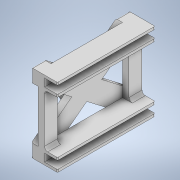
# Autodesk Inventor part: New_ThinGripper
Saved by Autodesk Inventor 2021 (Build 250183000, 183)
## iProperties
Created: 2021-08-05
Part Number: New_ThinGripper
Material: Generic
Document SubType Name: Modeling
Designer: hp
Density: 1 g/cm^3
Appearance: Default
Author: hp
Autodesk Inventor part; units mm, degrees
sketch "Sketch1" plane through (0, 0, 0) normal (1, 0, 0) x (0, 1, 0)
  circle A0 centre (0, 0) radius 2.5
  dimension "d0" = 5
  constraints: 1 centre point, 1 coincident
  measures "d0" diameter of A0
extrude "Extrusion1" add sketch "Sketch1" along normal blind 1
ref_plane "Work Plane1" through (1, 0, 0) normal (1, 0, 0) x (0, 0, -1)
sketch "Sketch2" plane through (1, 0, 0) normal (1, 0, 0) x (0, 0, -1)
  line L0 (-7.5, -6) -> (7.5, -6)
  line L1 (7.5, -6) -> (7.5, 6)
  line L2 (7.5, 6) -> (-7.5, 6)
  line L3 (-7.5, 6) -> (-7.5, -6)
  line L4 (-7.5, -6) -> (7.5, 6) construction
  line L5 (7.5, -6) -> (-7.5, 6) construction
  line L6 (7.5, 6) -> (5.5, 6)
  line L7 (7.5, 6) -> (7.5, 4)
  line L8 (7.5, -6) -> (7.5, -4)
  line L9 (7.5, -6) -> (5.5, -6)
  line L10 (-7.5, -6) -> (-5.5, -6)
  line L11 (-7.5, 6) -> (-7.5, 4)
  line L12 (-7.5, 6) -> (-5.5, 6)
  line L13 (-7.5, -6) -> (-7.5, -4)
  line L14 (-7.5, -4) -> (5.5, 6)
  line L15 (-5.5, -6) -> (7.5, 4)
  line L16 (-5.5, 6) -> (7.5, -4)
  line L17 (-7.5, 4) -> (5.5, -6)
  point P0 (0, 0)
  point P1 (-2.3, 0)
  point P2 (0, -1.7692)
  point P3 (2.3, 0)
  point P4 (0, 1.7692)
  dimension "d4" = 15
  dimension "d5" = 12
  dimension "d6" = 2
  dimension "d7" = 2
  dimension "d8" = 2
  dimension "d9" = 2
  dimension "d10" = 2
  dimension "d11" = 2
  dimension "d12" = 2
  dimension "d13" = 2
  constraints: 36 end point, 8 point on line, 2 midpoint, 2 parallel, 1 horizontal, 1 perpendicular
  measures "d4" distance of L0.start L0.end
  measures "d5" distance of L1.end L0.end
  measures "d6" distance of L1.end L6.end
  measures "d7" distance of L1.end L7.end
  measures "d8" distance of L0.end L8.end
  measures "d9" distance of L0.end L9.end
  measures "d10" distance of L0.start L10.end
  measures "d11" distance of L2.end L11.end
  measures "d12" distance of L2.end L12.end
  measures "d13" distance of L0.start L13.end
extrude "Extrusion2" add sketch "Sketch2" along normal blind 1 contours L3 L14 L17 L15 L0 | L17 L15 L16 L1 L0 | L17 L14 L16 L15 | L3 L2 L16 L14 L17 | L16 L14 L2 L1 L15
ref_plane "Work Plane2" through (2, 0, 0) normal (1, 0, 0) x (0, 0, -1)
sketch "Sketch3" plane through (2, 0, 0) normal (1, 0, 0) x (0, 0, -1)
  line L0 (-5.5, 6) -> (-7.5, 6) projected
  line L1 (-7.5, 6) -> (7.5, 6)
  line L2 (5.5, -6) -> (7.5, -6) projected
  line L3 (7.5, 6) -> (7.5, -6)
  line L4 (-7.5, -6) -> (-5.5, -6) projected
  line L5 (7.5, -6) -> (-7.5, -6)
  line L6 (-7.5, -6) -> (-7.5, 6)
  line L7 (-7.5, 4) -> (-2.4955, 0.1504) projected
  line L8 (2.4955, 0.1504) -> (7.5, 4) projected
  line L9 (-7.5, 4) -> (7.5, 4)
  line L10 (-2.3, 0) -> (-7.5, -4) projected
  line L11 (-7.5, -4) -> (7.5, -4)
  line L12 (-0.7854, 2.3734) -> (-5.5, 6) projected
  line L13 (-5.5, 6) -> (-5.5, -6)
  line L14 (0, -1.7692) -> (5.5, -6) projected
  line L15 (5.5, 6) -> (0, 1.7692) projected
  line L16 (5.5, -6) -> (5.5, 6)
  point P0 (0, 0)
  point P1 (-5.5, 4)
  point P2 (5.5, 4)
  point P3 (5.5, -4)
  point P4 (-5.5, -4)
  dimension "d17" = 15
  constraints: 16 end point, 2 horizontal, 2 perpendicular, 2 vertical, 1 collinear, 1 point on line
  measures "d17" distance of L0.end L1.end
extrude "Extrusion3" add sketch "Sketch3" along normal blind 1 contours L13 L9 L6 L0 | L1 L15 L9 L12 | L12 L9 L13 | L16 L9 L15 | L1 L3 L9 L16 | L13 L7 L9 | L7 L13 L10 L6 | L9 L8 L16 | L11 L13 L4 L6 | L10 L13 L11 | L3 L11 L16 L8 | L11 L14 L5 L13 | L3 L2 L16 L11 | L16 L14 L11
ref_plane "Work Plane3" through (3, 0, 0) normal (1, 0, 0) x (0, 0, -1)
sketch "Sketch4" plane through (3, 0, 0) normal (1, 0, 0) x (0, 0, -1)
  line L0 (7.5, 6) -> (-7.5, 6) projected
  line L1 (-7.5, 6) -> (7.5, 6)
  line L2 (7.5, 6) -> (7.5, 5.6)
  line L3 (7.5, 5.6) -> (-7.5, 5.6)
  line L4 (-7.5, 5.6) -> (-7.5, 6)
  line L5 (-7.5, 6) -> (-7.5, 4) projected
  line L6 (7.5, -4) -> (7.5, 4) projected
  line L7 (-7.5, 4) -> (7.5, 4)
  line L8 (7.5, 4) -> (7.5, 4.4)
  line L9 (7.5, 4.4) -> (-7.5, 4.4)
  line L10 (-7.5, 4.4) -> (-7.5, 4)
  line L11 (-7.5, -4) -> (-7.5, -6) projected
  line L12 (-7.5, -4) -> (7.5, -4)
  line L13 (7.5, -4) -> (7.5, -4.4)
  line L14 (7.5, -4.4) -> (-7.5, -4.4)
  line L15 (-7.5, -4.4) -> (-7.5, -4)
  line L16 (7.5, -6) -> (7.5, 6) projected
  line L17 (-7.5, -6) -> (7.5, -6)
  line L18 (7.5, -6) -> (7.5, -5.6)
  line L19 (7.5, -5.6) -> (-7.5, -5.6)
  line L20 (-7.5, -5.6) -> (-7.5, -6)
  point P0 (0, 0)
  dimension "d21" = 0.4
  dimension "d22" = 0.4
  dimension "d23" = 0.4
  dimension "d24" = 0.4
  constraints: 32 end point, 8 parallel, 7 perpendicular, 1 horizontal, 1 point on line
  measures "d21" distance of L0.start L2.end
  measures "d22" distance of L8.end L6.end
  measures "d23" distance of L6.start L13.end
  measures "d24" distance of L18.end L16.start
extrude "Extrusion4" add sketch "Sketch4" along normal blind 2 contours L2 L3 L4 L0 | L8 L7 L5 L9 | L12 L13 L14 L11 | L19 L16 L17 L11
fillet "Fillet1" radius 0.2 8 edges at (1, 6, 6.5) (1, 5, 7.5) (1, -5, 7.5) (1, -6, 6.5) (1, -6, -6.5) (1, -5, -7.5) (1, 5, -7.5) (1, 6, -6.5)
fillet "Fillet2" radius 0.1 4 edges at (1, -1.5243, 1.9816) (1, 1.5243, -1.9816) (1, 1.5243, 1.9816) (1, -1.5243, -1.9816)
fillet "Fillet3" radius 0.2 8 edges at (5, 5.8, -7.5) (5, 4.2, -7.5) (5, 5.8, 7.5) (5, 4.2, 7.5) (5, -4.2, 7.5) (5, -5.8, 7.5) (5, -5.8, -7.5) (5, -4.2, -7.5)
fillet "Fillet4" radius 0.5 4 edges at (3, 4, 6.5) (3, -4, 6.5) (3, 4, -6.5) (3, -4, -6.5)
body "Solid1"
